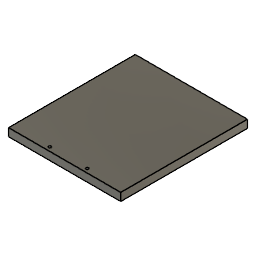
leftside (Autodesk Fusion 360 design; units mm, degrees)
Autodesk Fusion 360 part; units mm, degrees
sketch "Skizze1" plane through (0, 0, 0) normal (0, 0, 1) x (1, 0, 0)
  line L0 (127, 0) -> (127, 143.5)
  line L1 (0, 143.5) -> (0, 0)
  line L2 (0, 0) -> (127, 0)
  circle A0 centre (84.6667, 4.5) radius 1.5
  circle A1 centre (42.3337, 4.5) radius 1.5
  line L3 (127, 143.5) -> (0, 143.5)
  dimension "d1" = 127
  dimension "d2" = 143.5
  dimension "d7" = 3
  dimension "d8" = 4.5
  dimension "d9" = 42.3333
  dimension "d10" = 3
  constraint horizontal L2
  constraint vertical L0
  constraint horizontal L3
  constraint vertical L1
  constraint coincident L1.end L2.start
  measures "d1" distance of L0.start L1.end
  measures "d2" distance of L1.end L1.start
  measures "d7" diameter of A0
  measures "d8" distance of A0.centre L2
  measures "d9" distance of A0.centre L0
  measures "d10" diameter of A1
extrude "Extrusion1" add sketch "Skizze1" along normal blind 9
